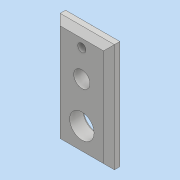
# Autodesk Inventor part: P5
Saved by Autodesk Inventor 2017 (Build 210142000, 142)
## iProperties
Part Number: P5
Material: 一般
Document SubType Name: Modeling
Designer: d8910
Density: 1 g/cm^3
Appearance: 預設
Author: d8910
Autodesk Inventor part; units mm, degrees
ref_plane "YZ Plane" through (0, 0, 0) normal (1, 0, 0) x (0, 1, 0)
ref_plane "XZ Plane" through (0, 0, 0) normal (0, 1, 0) x (-1, 0, 0)
ref_plane "XY Plane" through (0, 0, 0) normal (0, 0, 1) x (1, 0, 0)
sketch "草圖1" plane through (0, 0, 0) normal (0, 1, 0) x (-1, 0, 0)
  line L0 (50, 100) -> (-50, 100)
  line L1 (-50, 100) -> (-50, -100)
  line L2 (-50, -100) -> (50, -100)
  line L3 (50, -100) -> (50, 100)
  point P0 (0, 0)
  point P1 (0, 100)
  point P2 (50, 0)
  dimension "d0" = 200
  dimension "d1" = 100
  constraints: 8 end point, 2 midpoint, 2 parallel, 1 horizontal, 1 horizontal alignment, 1 perpendicular, 1 vertical alignment
  measures "d0" distance of L2.end L0.start
  measures "d1" distance of L0.start L0.end
extrude "擠出1" add sketch "草圖1" along normal mid plane 30
chamfer "倒角1" distance 10 angle 45 8 edges at (50, 15, 0) (0, 15, 100) (-50, 15, 0) (0, 15, -100) (0, -15, -100) (50, -15, 0) (-50, -15, 0) (0, -15, 100)
sketch "草圖2" plane through (0, 15, 0) normal (0, 1, 0) x (1, 0, 0)
  line L0 (-40, -90) -> (-40, 90) construction
  line L1 (40, -90) -> (-40, -90) construction
  line L2 (40, 90) -> (40, -90) construction
  line L3 (-40, 90) -> (40, 90) construction
  circle A0 centre (0, 50) radius 22.5
  circle A1 centre (0, -25) radius 15
  circle A2 centre (0, -75) radius 7.5
  line L4 (-50, -100) -> (50, -100) projected
  point P0 (0, 0)
  dimension "d7" = 45
  dimension "d8" = 30
  dimension "d9" = 15
  dimension "d10" = 25
  dimension "d11" = 50
  dimension "d12" = 75
  constraints: 3 centre point, 3 vertical alignment
  measures "d7" diameter of A0
  measures "d8" diameter of A1
  measures "d9" diameter of A2
  measures "d10" distance from line of L4 A2.centre
  measures "d11" distance of A1.centre A2.centre
  measures "d12" distance of A0.centre A1.centre
extrude "擠出2" cut sketch "草圖2" against normal through all
chamfer "倒角2" distance 5 angle 45 3 edges at (-7.5, 15, 75) (-15, 15, 25) (-22.5, 15, -50)
